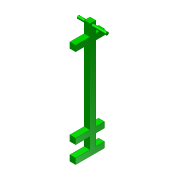
# Autodesk Inventor part: InnerTelescopeMockup
Saved by Autodesk Inventor 2012 (Build 160160000, 160)
## iProperties
Created: 2013-01-12
Part Number: InnerTelescopeMockup
Material: Default
Document SubType Name: Modeling
Designer: JesseK
Density: 1 g/cm^3
Author: JesseK
Autodesk Inventor part; units mm, degrees
ref_plane "YZ Plane" through (0, 0, 0) normal (1, 0, 0) x (0, 1, 0)
ref_plane "XZ Plane" through (0, 0, 0) normal (0, 1, 0) x (-1, 0, 0)
ref_plane "XY Plane" through (0, 0, 0) normal (0, 0, 1) x (1, 0, 0)
sketch "Sketch2" plane through (0, 0, 0) normal (0, 1, 0) x (-1, 0, 0)
  line L0 (0, 0) -> (25.4, 0)
  line L1 (25.4, 0) -> (25.4, 25.4)
  line L2 (25.4, 25.4) -> (0, 25.4)
  line L3 (0, 25.4) -> (0, 0)
  dimension "d0" = 25.4
  dimension "d1" = 25.4
  constraints: 8 end point, 2 parallel, 1 horizontal, 1 perpendicular
  measures "d0" distance of L2.end L0.start
  measures "d1" distance of L0.start L0.end
extrude "Extrusion1" add sketch "Sketch2" along normal blind 508
sketch "Sketch3" plane through (0, 0, 25.4) normal (1, 0, 0) x (0, 0, -1)
  line L0 (25.4, 508) -> (0, 508) projected
  line L1 (25.4, 0) -> (25.4, 508) projected
  circle A0 centre (12.7, 495.3) radius 6.35
  dimension "d4" = 12.7
  dimension "d5" = 12.7
  dimension "d6" = 12.7
  constraints: 1 centre point
  measures "d4" diameter of A0
  measures "d5" distance from line of L1 A0.centre
  measures "d6" distance from line of L0 A0.centre
extrude "Extrusion2" add sketch "Sketch3" along normal mid plane 127
sketch "Sketch4" plane through (-25.4, 0, 25.4) normal (0, 0, 1) x (1, 0, 0)
  line L0 (25.4, 508) -> (0, 508) projected
  line L1 (0, 0) -> (0, 508) projected
  line L2 (0, 0) -> (25.4, 0) projected
  line L3 (25.4, 0) -> (25.4, 508) projected
  line L4 (0, 457.2) -> (25.4, 457.2)
  line L5 (25.4, 457.2) -> (25.4, 431.8)
  line L6 (25.4, 431.8) -> (0, 431.8)
  line L7 (0, 431.8) -> (0, 457.2)
  line L8 (0, 101.6) -> (25.4, 101.6)
  line L9 (25.4, 101.6) -> (25.4, 76.2)
  line L10 (25.4, 76.2) -> (0, 76.2)
  line L11 (0, 76.2) -> (0, 101.6)
  line L12 (0, 0) -> (25.4, 0)
  line L13 (25.4, 0) -> (25.4, 25.4)
  line L14 (25.4, 25.4) -> (0, 25.4)
  line L15 (0, 25.4) -> (0, 0)
  dimension "d9" = 25.4
  dimension "d10" = 50.8
  dimension "d11" = 25.4
  dimension "d13" = 330.2
  dimension "d14" = 381
  dimension "d17" = 25.4
  dimension "d18" = 101.6
  constraints: 24 end point, 6 parallel, 6 point on line, 3 horizontal, 3 perpendicular
  measures "d9" distance of L5.end L4.end
  measures "d10" distance between parallel lines of L0 L4
  measures "d11" distance of L10.end L8.start
  measures "d13" distance between parallel lines of L8 L6
  measures "d14" distance between parallel lines of L10 L4
  measures "d17" distance of L14.end L1.start
  measures "d18" distance between parallel lines of L8 L2
extrude "Extrusion3" add sketch "Sketch4" along normal mid plane 127 contours L3 L6 L1 L4 | L3 L10 L1 L8 | L3 L2 L1 L14
body "Solid1"
